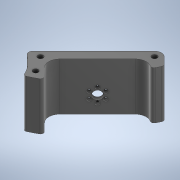
# Autodesk Inventor part: left_mount
Saved by Autodesk Inventor 2020 (Build 240168000, 168)
## iProperties
Created: 2023-12-16
Part Number: left_mount
Material: Пластмасса, непрозрачная, черная
Document SubType Name: Modeling
Designer: denis
Density: 0.952 g/cm^3
Appearance: Гладкая — черная
Author: denis
Autodesk Inventor part; units mm, degrees
ref_plane "YZ Plane" through (0, 0, 0) normal (1, 0, 0) x (0, 1, 0)
ref_plane "XZ Plane" through (0, 0, 0) normal (0, 1, 0) x (-1, 0, 0)
ref_plane "XY Plane" through (0, 0, 0) normal (0, 0, 1) x (1, 0, 0)
sketch "Эскиз1" plane through (0, 0, 0) normal (0, 1, 0) x (-1, 0, 0)
  line L0 (34.294679, -76.013979) -> (76.013979, -34.294679)
  arc A0 (83.085047, -34.294679) -> (76.013979, -34.294679) centre (79.549513, -37.830213) ccw
  line L1 (83.085047, -34.294679) -> (87.156031, -38.365663)
  line L2 (46.315494, -73.892659) -> (73.892659, -46.315494)
  arc A1 (85.206367, -46.315494) -> (73.892659, -46.315494) centre (79.549513, -51.972348) ccw
  line L3 (85.206367, -46.315494) -> (87.564456, -48.673583)
  line L4 (92.554343, -49.585216) -> (94.519181, -45.728813)
  line L5 (87.156031, -38.365663) -> (94.519181, -45.728813)
  line L6 (34.294679, -83.085047) -> (38.365663, -87.156031)
  arc A2 (34.294679, -76.013979) -> (34.294679, -83.085047) centre (37.830213, -79.549513) ccw
  arc A3 (46.315494, -73.892659) -> (46.315494, -85.206367) centre (51.972348, -79.549513) ccw
  line L7 (48.673583, -87.564456) -> (46.315494, -85.206367)
  line L8 (48.701386, -93.022443) -> (45.728813, -94.519181)
  line L9 (38.365663, -87.156031) -> (45.728813, -94.519181)
  spline S0 degree 4 poles (87.564456, -48.673583) (88.132682, -49.241799) (88.870839, -49.886462) (89.749506, -50.471004) (90.712651, -50.726306) (91.493885, -50.699943) (92.026144, -50.368221) (92.351861, -49.94776) (92.554343, -49.585216) knots 0 0 0 0 0 0.37630011 0.50133526 0.61466649 0.72228726 1 1 1 1 1
  spline S1 degree 4 poles (48.673583, -87.564456) (49.219633, -88.111097) (49.831751, -88.837474) (50.355302, -89.735854) (50.492035, -90.763763) (50.317855, -91.67706) (49.798776, -92.319536) (49.208663, -92.742933) (48.701386, -93.022443) knots 0 0 0 0 0 0.34950164 0.46930898 0.58208787 0.69415522 1 1 1 1 1
  line L10 (-34.294679, -83.085047) -> (-38.365663, -87.156031)
  arc A4 (-34.294679, -83.085047) -> (-34.294679, -76.013979) centre (-37.830213, -79.549513) ccw
  line L11 (-34.294679, -76.013979) -> (-76.013979, -34.294679)
  arc A5 (-76.013979, -34.294679) -> (-83.085047, -34.294679) centre (-79.549513, -37.830213) ccw
  line L12 (-83.085047, -34.294679) -> (-87.156031, -38.365663)
  spline S2 degree 4 poles (-87.564456, -48.673583) (-88.290466, -48.91192) (-89.207553, -49.153816) (-90.215753, -49.349229) (-91.17722, -49.491641) (-91.801106, -49.570889) (-92.194579, -49.603794) (-92.437828, -49.610977) (-92.554343, -49.585216) knots 0 0 0 0 0 0.41816963 0.55803166 0.68104119 0.78839296 1 1 1 1 1
  line L13 (-85.206367, -46.315494) -> (-87.564456, -48.673583)
  arc A6 (-73.892659, -46.315494) -> (-85.206367, -46.315494) centre (-79.549513, -51.972348) ccw
  line L14 (-46.315494, -73.892659) -> (-73.892659, -46.315494)
  arc A7 (-46.315494, -85.206367) -> (-46.315494, -73.892659) centre (-51.972348, -79.549513) ccw
  spline S3 degree 4 poles (-48.673583, -87.564456) (-49.219633, -88.111097) (-49.831751, -88.837474) (-50.355302, -89.735854) (-50.492035, -90.763763) (-50.317855, -91.67706) (-49.798776, -92.319536) (-49.208663, -92.742933) (-48.701386, -93.022443) knots 0 0 0 0 0 0.34950164 0.46930898 0.58208787 0.69415522 1 1 1 1 1
  line L15 (-48.673583, -87.564456) -> (-46.315494, -85.206367)
  arc A8 (-92.554343, 49.585216) -> (-92.554343, -49.585216) centre (0, 0) ccw construction
  arc A9 (-48.701386, -93.022443) -> (48.701386, -93.022443) centre (0, 0) ccw construction
  line L16 (-38.365663, -87.156031) -> (-45.728813, -94.519181)
  line L17 (-87.156031, -38.365663) -> (-94.519181, -45.728813)
  line L18 (-92.554343, -49.585216) -> (-94.519181, -45.728813)
  line L19 (-48.701386, -93.022443) -> (-45.728813, -94.519181)
  line L20 (0, 0) -> (0, 95.32372) construction
  line L21 (34.294679, -76.013979) -> (76.013979, -34.294679)
  arc A10 (83.085047, -34.294679) -> (76.013979, -34.294679) centre (79.549513, -37.830213) ccw
  line L22 (83.085047, -34.294679) -> (87.156031, -38.365663)
  line L23 (46.315494, -73.892659) -> (73.892659, -46.315494)
  arc A11 (85.206367, -46.315494) -> (73.892659, -46.315494) centre (79.549513, -51.972348) ccw
  line L24 (85.206367, -46.315494) -> (87.564456, -48.673583)
  line L25 (92.554343, -49.585216) -> (94.519181, -45.728813)
  arc A12 (92.554343, -49.585216) -> (92.554343, 49.585216) centre (0, 0) ccw construction
  line L26 (87.156031, -38.365663) -> (94.519181, -45.728813)
  line L27 (34.294679, -83.085047) -> (38.365663, -87.156031)
  arc A13 (34.294679, -76.013979) -> (34.294679, -83.085047) centre (37.830213, -79.549513) ccw
  arc A14 (46.315494, -73.892659) -> (46.315494, -85.206367) centre (51.972348, -79.549513) ccw
  line L28 (48.673583, -87.564456) -> (46.315494, -85.206367)
  line L29 (48.701386, -93.022443) -> (45.728813, -94.519181)
  line L30 (38.365663, -87.156031) -> (45.728813, -94.519181)
  arc A15 (-48.701386, -93.022443) -> (48.701386, -93.022443) centre (0, 0) ccw construction
  spline S4 degree 4 poles (87.564456, -48.673583) (88.132682, -49.241799) (88.870839, -49.886462) (89.749506, -50.471004) (90.712651, -50.726306) (91.493885, -50.699943) (92.026144, -50.368221) (92.351861, -49.94776) (92.554343, -49.585216) knots 0 0 0 0 0 0.37630011 0.50133526 0.61466649 0.72228726 1 1 1 1 1
  spline S5 degree 4 poles (48.673583, -87.564456) (49.219633, -88.111097) (49.831751, -88.837474) (50.355302, -89.735854) (50.492035, -90.763763) (50.317855, -91.67706) (49.798776, -92.319536) (49.208663, -92.742933) (48.701386, -93.022443) knots 0 0 0 0 0 0.34950164 0.46930898 0.58208787 0.69415522 1 1 1 1 1
  line L31 (52.209117, 91.09999) -> (48.673583, 87.564456) construction
  line L32 (52.209117, 91.09999) -> (48.673583, 87.564456) construction
  line L33 (48.673583, 87.564456) -> (52.209117, 91.09999) construction
  spline S6 degree 2 poles (48.673583, 87.564456) (52.209117, 91.09999) (48.701386, 93.022443) knots 1 1 1 2 2 2 construction
  line L34 (52.209117, 91.09999) -> (48.701386, 93.022443) construction
  line L35 (91.09999, 52.209117) -> (52.209117, 91.09999) construction
  arc A16 (92.554343, 49.585216) -> (48.701386, 93.022443) centre (0, 0) ccw construction
  line L36 (44.194174, 76.013979) -> (76.013979, 44.194174) construction
  line L37 (0, 56.641829) -> (-35.551578, 86.474449) construction
  arc A17 (0, 67.941027) -> (23.782532, 76.596871) centre (0, 104.941027) ccw construction
  arc A18 (-23.782532, 76.596871) -> (0, 67.941027) centre (0, 104.941027) ccw construction
  line L38 (-23.782532, 76.596871) -> (-35.273406, 86.238438) construction
  line L39 (0, 104.941) -> (-23.602791, 54.324652) construction
  arc A19 (-28.019871, 71.016304) -> (5.541335, 61.291358) centre (0, 104.941027) ccw construction
  arc A20 (5.541335, 61.291358) -> (28.019871, 71.016304) centre (0, 104.941027) ccw construction
  arc A21 (-30.639333, 73.21439) -> (-37.388887, 72.919771) centre (-33.853353, 69.384237) ccw construction
  line L40 (0, 56.641829) -> (23.782532, 76.596871) construction
  line L41 (23.782532, 76.596871) -> (35.273406, 86.238438) construction
  line L42 (0, 0) -> (74.246212, 74.246212) construction
  line L43 (42.6652, 95.941027) -> (42.049178, 94.573359) construction
  line L44 (42.049178, 94.573359) -> (42.6652, 95.941027) construction
  spline S7 degree 2 poles (42.049178, 94.573359) (42.6652, 95.941027) (43.576979, 95.530345) knots 1 1 1 2 2 2 construction
  line L45 (42.6652, 95.941027) -> (43.576979, 95.530345) construction
  arc A22 (-44.194174, 76.013979) -> (-44.194174, 83.085047) centre (-47.729708, 79.549513) ccw construction
  arc A23 (92.554343, -49.585216) -> (92.554343, 49.585216) centre (0, 0) ccw construction
  circle A24 centre (0, 0) radius 35 construction
  spline S8 degree 2 poles (-48.673583, 87.564456) (-52.209117, 91.09999) (-48.701386, 93.022443) knots 1 1 1 2 2 2 construction
  line L46 (-48.673583, 87.564456) -> (-52.209117, 91.09999) construction
  line L47 (-52.209117, 91.09999) -> (-48.701386, 93.022443) construction
  arc A25 (-83.085047, 44.194174) -> (-76.013979, 44.194174) centre (-79.549513, 47.729708) ccw construction
  line L48 (-83.085047, 44.194174) -> (-85.206367, 46.315494) construction
  line L49 (-44.194174, 76.013979) -> (-46.315494, 73.892659) construction
  arc A26 (-48.701386, 93.022443) -> (-92.554343, 49.585216) centre (0, 0) ccw construction
  line L50 (-42.6652, 95.941027) -> (-42.049178, 94.573359) construction
  arc A27 (-43.576979, 95.530345) -> (-48.701386, 93.022443) centre (0, 0) ccw
  ellipse E0 centre (0, 102.751067) end of major axis (-44.515859, 105.244484) minor radius 28.886984 (-42.049178, 94.573359) -> (-35.273406, 86.238438) ccw
  line L51 (-42.049178, 94.573359) -> (-42.6652, 95.941027) construction
  spline S9 degree 2 poles (-42.049178, 94.573359) (-42.6652, 95.941027) (-43.576979, 95.530345) knots 1 1 1 2 2 2 construction
  line L52 (-42.6652, 95.941027) -> (-43.576979, 95.530345) construction
  line L53 (-42.049178, 94.573359) -> (-42.6652, 95.941027) construction
  spline S10 degree 2 poles (-42.049178, 94.573359) (-42.6652, 95.941027) (-43.576979, 95.530345) knots 1 1 1 2 2 2
  line L54 (-42.6652, 95.941027) -> (-43.576979, 95.530345) construction
  line L55 (-42.6652, 95.941027) -> (-43.576979, 95.530345) construction
  line L56 (-44.194174, 83.085047) -> (-48.673583, 87.564456) construction
  line L57 (-37.388887, 72.919771) -> (-76.013979, 34.294679)
  arc A28 (-83.085047, 34.294679) -> (-76.013979, 34.294679) centre (-79.549513, 37.830213) ccw
  line L58 (-83.085047, 34.294679) -> (-90.689075, 41.898707)
  arc A29 (-87.35626, 48.465387) -> (-90.689075, 41.898707) centre (0, 0) ccw construction
  line L59 (-93.52971, 47.670855) -> (-92.554343, 49.585216) construction
  arc A30 (85.206367, -46.315494) -> (73.892659, -46.315494) centre (79.549513, -51.972348) ccw construction
  line L60 (85.206367, -46.315494) -> (87.564456, -48.673583) construction
  spline S11 degree 2 poles (87.564456, -48.673583) (91.09999, -52.209117) (92.554343, -49.585216) knots 1 1 1 2 2 2 construction
  line L61 (87.564456, -48.673583) -> (91.09999, -52.209117) construction
  line L62 (91.09999, -52.209117) -> (92.554343, -49.585216) construction
  line L63 (46.315494, -73.892659) -> (73.892659, -46.315494) construction
  line L64 (48.673583, -87.564456) -> (46.315494, -85.206367) construction
  line L65 (48.673583, -87.564456) -> (52.209117, -91.09999) construction
  spline S12 degree 2 poles (48.673583, -87.564456) (52.209117, -91.09999) (48.701386, -93.022443) knots 1 1 1 2 2 2 construction
  line L66 (52.209117, -91.09999) -> (48.701386, -93.022443) construction
  arc A31 (46.315494, -73.892659) -> (46.315494, -85.206367) centre (51.972348, -79.549513) ccw construction
  arc A32 (48.701386, -93.022443) -> (92.554343, -49.585216) centre (0, 0) ccw construction
  arc A33 (-48.701386, -93.022443) -> (48.701386, -93.022443) centre (0, 0) ccw construction
  arc A34 (-90.689075, 41.898707) -> (-87.35626, 48.465387) centre (0, 0) ccw construction
  line L67 (42.6652, 95.941027) -> (-42.6652, 95.941027) construction
  line L68 (-48.673583, -87.564456) -> (-52.209117, -91.09999) construction
  spline S13 degree 2 poles (-48.673583, -87.564456) (-52.209117, -91.09999) (-48.701386, -93.022443) knots 1 1 1 2 2 2 construction
  line L69 (-52.209117, -91.09999) -> (-48.701386, -93.022443) construction
  line L70 (-91.09999, -52.209117) -> (-92.554343, -49.585216) construction
  spline S14 degree 2 poles (-87.564456, -48.673583) (-91.09999, -52.209117) (-92.554343, -49.585216) knots 1 1 1 2 2 2 construction
  line L71 (-87.564456, -48.673583) -> (-91.09999, -52.209117) construction
  arc A35 (-92.554343, -49.585216) -> (-48.701386, -93.022443) centre (0, 0) ccw construction
  line L72 (-48.673583, -87.564456) -> (-46.315494, -85.206367) construction
  arc A36 (-73.892659, -46.315494) -> (-85.206367, -46.315494) centre (-79.549513, -51.972348) ccw construction
  line L73 (-85.206367, -46.315494) -> (-87.564456, -48.673583) construction
  line L74 (-46.315494, -73.892659) -> (-73.892659, -46.315494) construction
  arc A37 (-46.315494, -85.206367) -> (-46.315494, -73.892659) centre (-51.972348, -79.549513) ccw construction
  arc A38 (-92.554343, 49.585216) -> (-92.554343, -49.585216) centre (0, 0) ccw construction
  arc A39 (44.194174, 83.085047) -> (44.194174, 76.013979) centre (47.729708, 79.549513) ccw construction
  arc A40 (44.027132, 95.32372) -> (43.576979, 95.530345) centre (0, 0) ccw construction
  line L75 (42.6652, 95.941027) -> (43.576979, 95.530345) construction
  arc A41 (48.701386, 93.022443) -> (44.027132, 95.32372) centre (0, 0) ccw construction
  line L76 (52.209117, 91.09999) -> (48.701386, 93.022443) construction
  line L77 (83.085047, 44.194174) -> (87.564456, 48.673583) construction
  ellipse E1 centre (0, 102.751067) end of major axis (44.515859, 105.244484) minor radius 28.886984 (35.273406, 86.238438) -> (42.049178, 94.573359) ccw construction
  arc A42 (76.013979, 44.194174) -> (83.085047, 44.194174) centre (79.549513, 47.729708) ccw construction
  line L78 (0, 0) -> (0, 209.882054) construction
  arc A43 (43.576979, 95.530345) -> (-43.576979, 95.530345) centre (0, 0) ccw construction
  arc A44 (23.782532, 76.596871) -> (0, 67.941027) centre (0, 104.941027) ccw construction
  line L79 (44.027132, 95.32372) -> (44.027132, 127.81619) construction
  ellipse E2 centre (0, 102.751067) end of major axis (44.027132, 102.751067) minor radius 27.593201 (42.049178, 94.573359) -> (35.273406, 86.238438) ccw construction
  line L80 (-30.639333, 73.21439) -> (-28.019871, 71.016304) construction
  arc A45 (28.019871, 71.016304) -> (-28.019871, 71.016304) centre (0, 104.941027) ccw construction
  line L81 (30.639333, 73.21439) -> (28.019871, 71.016304) construction
  arc A46 (37.388887, 72.919771) -> (30.639333, 73.21439) centre (33.853353, 69.384237) ccw construction
  line L82 (44.027132, 95.32372) -> (43.576979, 95.530345) construction
  arc A47 (44.194174, 83.085047) -> (44.194174, 76.013979) centre (47.729708, 79.549513) ccw construction
  line L83 (48.673583, 87.564456) -> (44.194174, 83.085047) construction
  line L84 (37.388887, 72.919771) -> (76.013979, 34.294679) construction
  line L85 (44.194174, 76.013979) -> (76.013979, 44.194174) construction
  arc A48 (76.013979, 44.194174) -> (83.085047, 44.194174) centre (79.549513, 47.729708) ccw construction
  arc A49 (76.013979, 34.294679) -> (83.085047, 34.294679) centre (79.549513, 37.830213) ccw construction
  line L86 (83.085047, 44.194174) -> (87.35626, 48.465387) construction
  line L87 (83.085047, 34.294679) -> (90.689075, 41.898707) construction
  arc A50 (90.689075, 41.898707) -> (87.35626, 48.465387) centre (0, 0) ccw construction
  arc A51 (-83.085047, 34.294679) -> (-76.013979, 34.294679) centre (-79.549513, 37.830213) ccw
  line L88 (-87.156031, 38.365663) -> (-94.519181, 45.728813)
  line L89 (-93.022443, 48.701386) -> (-94.519181, 45.728813)
  arc A52 (-85.206367, 46.315494) -> (-73.892659, 46.315494) centre (-79.549513, 51.972348) ccw
  line L90 (-87.564456, 48.673583) -> (-85.206367, 46.315494)
  line L91 (-83.085047, 34.294679) -> (-87.156031, 38.365663)
  line L92 (-73.892659, 46.315494) -> (-46.315494, 73.892659)
  spline S15 degree 4 poles (-87.564456, 48.673583) (-88.111097, 49.219633) (-88.837474, 49.831751) (-89.735854, 50.355302) (-90.763763, 50.492035) (-91.67706, 50.317855) (-92.319536, 49.798776) (-92.742933, 49.208663) (-93.022443, 48.701386) knots 0 0 0 0 0 0.34950164 0.46930898 0.58208787 0.69415522 1 1 1 1 1
  arc A53 (-34.294679, 76.013979) -> (-34.294679, 83.085047) centre (-37.830213, 79.549513) ccw construction
  line L93 (-34.294679, 83.085047) -> (-38.365663, 87.156031) construction
  arc A54 (-46.315494, 73.892659) -> (-46.315494, 85.206367) centre (-51.972348, 79.549513) ccw
  line L94 (-46.315494, 85.206367) -> (-48.673583, 87.564456)
  spline S16 degree 4 poles (-48.673583, 87.564456) (-49.241799, 88.132682) (-49.886462, 88.870839) (-50.471004, 89.749506) (-50.726306, 90.712651) (-50.699943, 91.493885) (-50.368221, 92.026144) (-49.94776, 92.351861) (-49.585216, 92.554343) knots 0 0 0 0 0 0.37630011 0.50133526 0.61466649 0.72228726 1 1 1 1 1
  line L95 (-49.585216, 92.554343) -> (-45.728813, 94.519181)
  line L96 (-38.365663, 87.156031) -> (-45.728813, 94.519181) construction
  arc A55 (-34.294679, 76.013979) -> (-34.294679, 83.085047) centre (-37.830213, 79.549513) ccw construction
  line L97 (-34.294679, 83.085047) -> (-38.365663, 87.156031) construction
  arc A56 (-46.315494, 73.892659) -> (-46.315494, 85.206367) centre (-51.972348, 79.549513) ccw
  line L98 (-46.315494, 85.206367) -> (-48.673583, 87.564456)
  spline S17 degree 4 poles (-48.673583, 87.564456) (-49.241799, 88.132682) (-49.886462, 88.870839) (-50.471004, 89.749506) (-50.726306, 90.712651) (-50.699943, 91.493885) (-50.368221, 92.026144) (-49.94776, 92.351861) (-49.585216, 92.554343) knots 0 0 0 0 0 0.37630011 0.50133526 0.61466649 0.72228726 1 1 1 1 1
  line L99 (-49.585216, 92.554343) -> (-45.728813, 94.519181)
  line L100 (-38.365663, 87.156031) -> (-45.728813, 94.519181) construction
  arc A57 (-83.085047, 34.294679) -> (-76.013979, 34.294679) centre (-79.549513, 37.830213) ccw
  line L101 (-83.085047, 34.294679) -> (-87.156031, 38.365663)
  line L102 (-87.156031, 38.365663) -> (-94.519181, 45.728813)
  line L103 (-93.022443, 48.701386) -> (-94.519181, 45.728813)
  spline S18 degree 4 poles (-87.564456, 48.673583) (-88.111097, 49.219633) (-88.837474, 49.831751) (-89.735854, 50.355302) (-90.763763, 50.492035) (-91.67706, 50.317855) (-92.319536, 49.798776) (-92.742933, 49.208663) (-93.022443, 48.701386) knots 0 0 0 0 0 0.34950164 0.46930898 0.58208787 0.69415522 1 1 1 1 1
  arc A58 (-85.206367, 46.315494) -> (-73.892659, 46.315494) centre (-79.549513, 51.972348) ccw
  line L104 (-76.013979, 34.294679) -> (-34.294679, 76.013979) construction
  line L105 (-73.892659, 46.315494) -> (-46.315494, 73.892659)
  line L106 (-87.564456, 48.673583) -> (-85.206367, 46.315494)
  line L107 (-87.564456, 48.673583) -> (-91.09999, 52.209117) construction
  spline S19 degree 2 poles (-87.564456, 48.673583) (-91.09999, 52.209117) (-93.022443, 48.701386) knots 1 1 1 2 2 2 construction
  line L108 (-91.09999, 52.209117) -> (-93.022443, 48.701386) construction
  line L109 (-48.673583, 87.564456) -> (-52.209117, 91.09999) construction
  spline S20 degree 2 poles (-48.673583, 87.564456) (-52.209117, 91.09999) (-49.585216, 92.554343) knots 1 1 1 2 2 2 construction
  line L110 (-52.209117, 91.09999) -> (-49.585216, 92.554343) construction
  arc A59 (-49.585216, 92.554343) -> (-93.022443, 48.701386) centre (0, 0) ccw construction
  arc A60 (-46.315494, 73.892659) -> (-46.315494, 85.206367) centre (-51.972348, 79.549513) ccw construction
  line L111 (-46.315494, 85.206367) -> (-48.673583, 87.564456) construction
  line L112 (-73.892659, 46.315494) -> (-46.315494, 73.892659) construction
  arc A61 (-85.206367, 46.315494) -> (-73.892659, 46.315494) centre (-79.549513, 51.972348) ccw construction
  line L113 (-87.564456, 48.673583) -> (-85.206367, 46.315494) construction
  line L114 (-60.104076, 60.104076) -> (-55.154329, 55.154329) construction
  circle A62 centre (-79.549513, 37.830213) radius 1.9
  circle A63 centre (-37.830213, 79.549513) radius 1.9
  arc A64 (-34.995029, 78.26992) -> (-31.495417, 78.813241) centre (-33.616737, 80.934561) ccw construction
  arc A65 (-36.584452, 80.495622) -> (-34.995029, 78.26992) centre (-33.616737, 80.934561) ccw construction
  arc A66 (-31.768725, 83.29779) -> (-36.584452, 80.495622) centre (-33.616737, 80.934561) ccw construction
  arc A67 (-31.495417, 78.813241) -> (-31.768725, 83.29779) centre (-33.616737, 80.934561) ccw
  line L115 (-31.495417, 78.813241) -> (-29.181616, 81.127042) construction
  line L116 (-46.315494, 73.892659) -> (-73.892659, 46.315494)
  line L117 (-73.892659, 46.315494) -> (-76.013979, 44.194174) construction
  line L118 (-85.206367, 46.315494) -> (-87.35626, 48.465387)
  line L119 (-31.768725, 83.29779) -> (-35.273406, 86.238438)
  line L120 (99.9, 0) -> (-99.9, 0) construction
  line L121 (-31.495417, 78.813241) -> (-37.388887, 72.919771)
  point P0 (49.53848, -88.539709)
  point P1 (50.086642, -89.38926)
  point P2 (50.373998, -90.130422)
  point P3 (50.446849, -90.78614)
  point P4 (50.331332, -91.383317)
  point P5 (50.025175, -91.946822)
  point P6 (49.49818, -92.492202)
  point P7 (88.575929, -49.593743)
  point P8 (89.433786, -50.202448)
  point P9 (90.155898, -50.55286)
  point P10 (90.764436, -50.694833)
  point P11 (91.285778, -50.66646)
  point P12 (91.746685, -50.483809)
  point P13 (92.167172, -50.135229)
  point P14 (-49.53848, -88.539709)
  point P15 (-50.086642, -89.38926)
  point P16 (-50.373998, -90.130422)
  point P17 (-50.446849, -90.78614)
  point P18 (-50.331332, -91.383317)
  point P19 (-50.025175, -91.946822)
  point P20 (-49.49818, -92.492202)
  point P21 (-88.807705, -49.034398)
  point P22 (-89.822287, -49.262919)
  point P23 (-90.628053, -49.407064)
  point P24 (-91.254259, -49.499666)
  point P25 (-91.73586, -49.558865)
  point P26 (-92.104118, -49.592535)
  point P27 (-92.376668, -49.602317)
  point P28 (88.575929, -49.593743)
  point P29 (89.433786, -50.202448)
  point P30 (90.155898, -50.55286)
  point P31 (90.764436, -50.694833)
  point P32 (91.285778, -50.66646)
  point P33 (91.746685, -50.483809)
  point P34 (92.167172, -50.135229)
  point P35 (49.53848, -88.539709)
  point P36 (50.086642, -89.38926)
  point P37 (50.373998, -90.130422)
  point P38 (50.446849, -90.78614)
  point P39 (50.331332, -91.383317)
  point P40 (50.025175, -91.946822)
  point P41 (49.49818, -92.492202)
  point P42 (79.549513, 40.65864)
  point P43 (40.65864, 79.549513)
  point P44 (60.104076, 60.104076)
  point P45 (-23.542039, 76.396809)
  point P46 (-34.993484, 86.006132)
  point P47 (0, 95.941027)
  point P48 (-15.636865, 71.407634)
  point P49 (-13.281664, 58.64894)
  point P50 (-28.545172, 71.457103)
  point P51 (13.281664, 58.64894)
  point P52 (-87.564456, 48.673583)
  point P53 (0, 105)
  point P54 (-94.519181, 45.728813)
  point P55 (0, 95.941027)
  point P56 (-88.539709, 49.53848)
  point P57 (-89.38926, 50.086642)
  point P58 (-90.130422, 50.373998)
  point P59 (-90.78614, 50.446849)
  point P60 (-91.383317, 50.331332)
  point P61 (-91.946822, 50.025175)
  point P62 (-92.492202, 49.49818)
  point P63 (-49.593743, 88.575929)
  point P64 (-50.202448, 89.433786)
  point P65 (-50.55286, 90.155898)
  point P66 (-50.694833, 90.764436)
  point P67 (-50.66646, 91.285778)
  point P68 (-50.483809, 91.746685)
  point P69 (-50.135229, 92.167172)
  point P70 (-49.593743, 88.575929)
  point P71 (-50.202448, 89.433786)
  point P72 (-50.55286, 90.155898)
  point P73 (-50.694833, 90.764436)
  point P74 (-50.66646, 91.285778)
  point P75 (-50.483809, 91.746685)
  point P76 (-50.135229, 92.167172)
  point P77 (-88.539709, 49.53848)
  point P78 (-89.38926, 50.086642)
  point P79 (-90.130422, 50.373998)
  point P80 (-90.78614, 50.446849)
  point P81 (-91.383317, 50.331332)
  point P82 (-91.946822, 50.025175)
  point P83 (-92.492202, 49.49818)
  dimension "d63" = 44.58564
  dimension "d44" = 74
  dimension "d45" = 100
  dimension "d46" = 28
  dimension "d47" = 15
  dimension "d48" = 45
  dimension "d49" = 55
  dimension "d50" = 16.33484
  dimension "d51" = 27.5
  dimension "d52" = 5
  dimension "d53" = 5
  dimension "d54" = 1
  dimension "d55" = 1.5
  dimension "d56" = 1.5
  dimension "d57" = 1
  dimension "d58" = 4
  dimension "d59" = 70
  dimension "d60" = 85
  dimension "d61" = 105
  dimension "d62" = 1.36193
  dimension "d64" = 88
  dimension "d65" = 7
  dimension "d66" = 5
  dimension "d67" = 7
  dimension "d68" = 5
  dimension "d69" = 7
  dimension "d70" = 5
  dimension "d71" = 5.1
  dimension "d72" = 3.8
  dimension "d73" = 6
  constraints: 200 end point, 159 point on circle, 145 symmetric about line, 67 centre point, 28 coincident, 20 point on line, 18 tangent, 11 collinear, 8 parallel, 6 midpoint, 4 vertical, 3 perpendicular, 2 horizontal, 1 concentric, 1 equal radius, 182 other
  measures "d44" diameter of A44
  measures "d45" angle of L37 L40
  measures "d46" distance from line of L67 A18.end
  measures "d47" distance of L40.end L41.end
  measures "d48" angle of L78 L42
  measures "d49" distance of point (40.659, 79.55) point (79.55, 40.659)
  measures "d50" distance of L35.start point (79.55, 40.659)
  measures "d51" distance of point (40.659, 79.55) point (60.104, 60.104)
  measures "d52" radius of A39
  measures "d53" distance of L76.start L31.end
  measures "d54" distance of L43.start L45.end
  measures "d55" distance of L43.start L43.end
  measures "d56" distance of L55.start L51.start
  measures "d57" distance of L55.start L52.end
  measures "d58" distance of L76.start L34.end
  measures "d59" diameter of A24
  measures "d60" distance of point (60.104, 60.104) L78.start
  measures "d61" radius of A23
  measures "d62" distance from line of L79 L67.start
  measures "d64" diameter of A45
  measures "d65" distance between parallel lines of L48 L58
  measures "d66" radius of A25
  measures "d67" distance between parallel lines of L57 L49
  measures "d68" radius of A28
  measures "d69" distance between parallel lines of L37 L80
  measures "d70" radius of A21
  measures "d71" radial gap between concentric circles of A38 A34
  measures "d72" diameter of A62
  measures "d73" diameter of A64
extrude "Выдавливание10" add sketch "Эскиз1" along normal blind 35 contours S10 E0 L119 A67 L121 L57 A28 L58 L88 L89 S15 L90 A52 L92 A54 L94 S16 L95 A27
sketch "Эскиз6" plane through (31.495417, 0, 78.813241) normal (-0.7071068, 0, -0.7071068) x (-0.7071068, 0, 0.7071068)
  line L0 (-5.858754, 35) -> (-2.058754, 35) construction
  line L1 (-64.858754, 35) -> (-61.058754, 35) construction
  line L2 (-61.058754, 0) -> (-64.858754, 0) construction
  line L3 (-5.858754, 0) -> (-2.058754, 0) construction
  line L4 (-62.958754, 0) -> (-67.958754, 0) construction
  line L5 (-62.958754, 35) -> (-62.958754, 0) construction
  line L6 (-62.958754, 35) -> (0, 35) construction
  line L7 (-121.958754, 35) -> (-121.958754, 0) construction
  line L8 (-62.958754, 0) -> (0, 0) construction
  circle A0 centre (-33.458754, 12) radius 8.25
  circle A1 centre (-33.458754, 12) radius 5 construction
  circle A2 centre (-33.458754, 12) radius 3.2
  circle A3 centre (-33.458754, 17) radius 1.15
  line L9 (-33.458754, 12) -> (-33.458754, 35) construction
  line L10 (-13.958754, 35) -> (-52.958754, 35) construction
  circle A4 centre (-37.788881, 14.5) radius 1.15
  circle A5 centre (-37.788881, 9.5) radius 1.15
  circle A6 centre (-33.458754, 7) radius 1.15
  circle A7 centre (-29.128627, 9.5) radius 1.15
  circle A8 centre (-29.128627, 14.5) radius 1.15
  point P0 (-33.458754, 0)
  dimension "d82" = 10
  dimension "d80" = 59
  dimension "d81" = 16.5
  dimension "d83" = 6.4
  dimension "d84" = 2.3
  dimension "d87" = 360
  dimension "d96" = 12
  constraints: 8 centre point, 6 end point, 3 point on line, 2 coincident, 2 midpoint, 2 perpendicular, 1 vertical, 1 vertical alignment, 15 other
  measures "d80" distance between parallel lines of L7 L5
  measures "d81" diameter of A0
  measures "d83" diameter of A2
  measures "d84" diameter of A3
  measures "d96" distance from line of L8 A0.centre
extrude "Выдавливание13" cut sketch "Эскиз6" against normal mid plane 33.5 contours A2 | A3 | A4 | A5 | A6 | A7 | A8
extrude "Выдавливание14" cut sketch "Эскиз6" against normal blind 4
chamfer "Фаска3" distance 0.5 angle 45 6 edges at (60.9172, 17, 59.2909) (63.9791, 14.5, 56.229) (63.9791, 9.5, 56.229) (60.9172, 7, 59.2909) (57.8554, 9.5, 62.3528) (57.8554, 14.5, 62.3528)
sketch "Эскиз7" plane through (0, 35, 0) normal (0, 1, 0) x (1, 0, 0)
  circle A0 centre (0, 0) radius 97.5
  line L0 (82.968504, -51.21013) -> (104.633896, -55.74756)
  line L1 (104.633896, -55.74756) -> (90.787409, -35.551319)
  dimension "d97" = 195
  constraints: 4 end point, 2 point on circle, 1 centre point, 1 coincident
  measures "d97" diameter of A0
extrude "Выдавливание15" cut sketch "Эскиз7" against normal blind 41.5 contours A0 L1 L0
fillet "Сопряжение1" radius 2 2 edges at (85.5892, 17.5, 46.6983) (88.8777, 17.5, 40.0874)
sketch "Эскиз8" plane through (0, 35, 0) normal (0, 1, 0) x (1, 0, 0)
  arc A0 (88.29008, -41.365586) -> (87.893215, -39.102848) centre (86.479002, -40.517061) ccw construction
  line L0 (87.893215, -39.102848) -> (83.085047, -34.294679) construction
  arc A1 (83.085047, -34.294679) -> (76.013979, -34.294679) centre (79.549513, -37.830213) ccw construction
  line L1 (76.013979, -34.294679) -> (31.495417, -78.813241) construction
  arc A2 (31.495417, -78.813241) -> (31.768725, -83.29779) centre (33.616737, -80.934561) ccw construction
  line L2 (31.768725, -83.29779) -> (35.273406, -86.238438) construction
  ellipse E0 centre (0, -102.751067) end of major axis (-44.515859, -100.25765) minor radius 28.886984 (42.049178, -94.573359) -> (35.273406, -86.238438) ccw
  arc A3 (43.576979, -95.530345) -> (45.728813, -94.519181) centre (0, 0) ccw construction
  line L3 (45.728813, -94.519181) -> (49.585216, -92.554343) construction
  line L4 (48.673583, -87.564456) -> (46.315494, -85.206367) construction
  arc A4 (46.315494, -73.892659) -> (46.315494, -85.206367) centre (51.972348, -79.549513) ccw construction
  line L5 (46.315494, -73.892659) -> (73.892659, -46.315494) construction
  arc A5 (83.893336, -45.254372) -> (73.892659, -46.315494) centre (79.549513, -51.972348) ccw construction
  arc A6 (83.893336, -45.254372) -> (86.758963, -44.487441) centre (84.979291, -43.574878) ccw construction
  arc A7 (86.758963, -44.487441) -> (88.29008, -41.365586) centre (0, 0) ccw construction
  circle A8 centre (79.549513, -37.830213) radius 1.9 construction
  circle A9 centre (37.830213, -79.549513) radius 1.9 construction
  circle A10 centre (0, 0) radius 107 construction
  line L6 (48.673583, -87.564456) -> (46.315494, -85.206367) construction
  line L7 (46.315494, -85.206367) -> (51.810265, -90.701138)
  ellipse E1 centre (0, -102.751067) end of major axis (-44.515859, -100.25765) minor radius 28.886984 (42.049178, -94.573359) -> (35.273406, -86.238438) ccw construction
  arc A11 (42.932521, -96.366056) -> (42.049178, -94.573359) centre (15.821192, -108.611056) ccw
  arc A12 (44.929406, -97.109981) -> (51.355976, -93.86993) centre (0, 0) ccw
  arc A13 (42.932521, -96.366056) -> (44.929406, -97.109981) centre (44.299554, -95.748627) ccw
  arc A14 (51.355976, -93.86993) -> (51.810265, -90.701138) centre (50.396051, -92.115352) ccw
  line L8 (42.049178, -94.573359) -> (46.315494, -85.206367)
  point P0 (53.673474, -92.564346)
  dimension "d101" = 214
  dimension "d102" = 1.5
  dimension "d103" = 2
  constraints: 11 point on circle, 5 centre point, 4 end point, 4 tangent, 1 coincident, 1 collinear, 1 concentric, 1 point on line, 4 other
  measures "d101" diameter of A10
  measures "d102" radius of A13
  measures "d103" radius of A14
extrude "Выдавливание16" add sketch "Эскиз8" against normal up to surface (35 mm away)
sketch "Эскиз9" plane through (0, 35, 0) normal (0, 1, 0) x (1, 0, 0)
  circle A0 centre (79.549513, -37.830213) radius 1.9 construction
  circle A1 centre (37.830213, -79.549513) radius 1.9 construction
  arc A2 (42.932521, -96.366056) -> (42.26265, -94.979714) centre (15.821192, -108.611056) ccw construction
  arc A3 (42.932521, -96.366056) -> (44.929406, -97.109981) centre (44.299554, -95.748627) ccw construction
  arc A4 (44.929406, -97.109981) -> (51.355976, -93.86993) centre (0, 0) ccw construction
  arc A5 (51.355976, -93.86993) -> (51.810265, -90.701138) centre (50.396051, -92.115352) ccw construction
  line L0 (51.810265, -90.701138) -> (46.315494, -85.206367) construction
  arc A6 (46.315494, -73.892659) -> (46.315494, -85.206367) centre (51.972348, -79.549513) ccw construction
  line L1 (46.315494, -73.892659) -> (73.892659, -46.315494) construction
  arc A7 (83.893336, -45.254372) -> (73.892659, -46.315494) centre (79.549513, -51.972348) ccw construction
  arc A8 (83.893336, -45.254372) -> (86.758963, -44.487441) centre (84.979291, -43.574878) ccw construction
  arc A9 (86.758963, -44.487441) -> (88.29008, -41.365586) centre (0, 0) ccw construction
  arc A10 (88.29008, -41.365586) -> (87.893215, -39.102848) centre (86.479002, -40.517061) ccw construction
  line L2 (87.893215, -39.102848) -> (83.085047, -34.294679) construction
  arc A11 (83.085047, -34.294679) -> (76.013979, -34.294679) centre (79.549513, -37.830213) ccw construction
  line L3 (76.013979, -34.294679) -> (31.495417, -78.813241) construction
  arc A12 (31.495417, -78.813241) -> (31.768725, -83.29779) centre (33.616737, -80.934561) ccw construction
  line L4 (31.768725, -83.29779) -> (35.273406, -86.238438) construction
  ellipse E0 centre (0, -102.751067) end of major axis (-44.515859, -100.25765) minor radius 28.886984 (42.049178, -94.573359) -> (35.273406, -86.238438) ccw construction
  circle A13 centre (0, 0) radius 101 construction
  circle A14 centre (45.111051, -90.365885) radius 1.9
  dimension "d106" = 202
  dimension "d107" = 3.8
  dimension "d108" = 4.5
  constraints: 1 centre point, 1 coincident, 5 other
  measures "d107" diameter of A14
  measures "d108" distance from line of L0 A14.centre
extrude "Выдавливание17" cut sketch "Эскиз9" against normal up to surface (35 mm away)
sketch "Эскиз10" plane through (0, 35, 0) normal (0, 1, 0) x (1, 0, 0)
  line L0 (86.995839, -35.5) -> (35.301185, -35.5)
  line L1 (35.301185, -35.5) -> (35.301185, 35.5)
  line L2 (35.301185, 35.5) -> (86.995839, 35.5)
  line L3 (86.995839, 35.5) -> (86.995839, -35.5)
  line L4 (0, 0) -> (115.972054, 0) construction
  dimension "d111" = 71
  constraints: 10 end point, 2 horizontal, 2 parallel, 1 perpendicular, 1 other
  measures "d111" distance of L0.end L1.end
sketch "Эскиз11" plane through (0, 0, 0) normal (0, -1, 0) x (1, 0, 0)
  line L0 (86.995839, 35.5) -> (35.301185, 35.5)
  line L1 (35.301185, 35.5) -> (35.301185, -35.5)
  line L2 (86.995839, -35.5) -> (86.995839, 35.5)
  line L3 (35.301185, -35.5) -> (86.995839, -35.5)
  point P0 (0, 0)
extrude "Выдавливание18" cut sketch "Эскиз11" against normal blind 23
chamfer "Фаска4" distance 2.5 angle 45 3 edges at (79.5495, 23, 32.8302) (75.4113, 23, 34.8973) (83.6877, 23, 34.8973)
